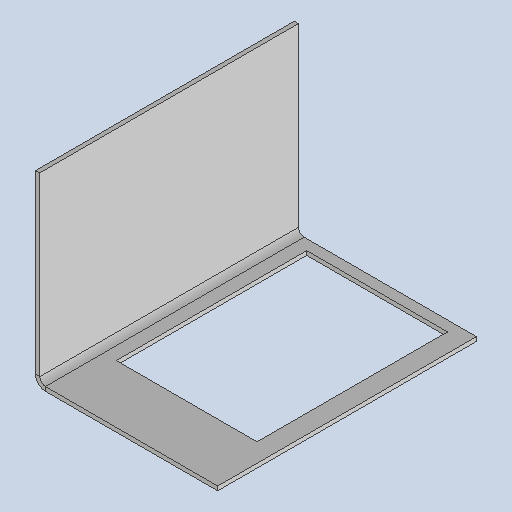
# Autodesk Inventor part: KND-1652 DrSysB Central tube wall 01
Saved by Autodesk Inventor 2026.2 (Build 302298000, 298)
## iProperties
Created: 2025-06-24
Part Number: KND-1652 DrSysB Central tube wall 01
Material: Stainless Steel
Document SubType Name: Sheet Metal
Designer: admin
Mass: 193.508 g
Surface Area: 260.557 cm^2
Volume: 24.1885 cm^3
Density: 8 g/cm^3
Flat Pattern Width: 17.4202 cm
Flat Pattern Length: 12.5 cm
Flat Pattern Area: 217.752 cm^2
Sheet Metal Rule: AISI304 2mm Die16
Sheet Metal Width: 174,202 mm
Sheet Metal Length: 125,000 mm
Sheet Metal Area: 21775,249 mm^2
Appearance: Default
Author: user
Autodesk Inventor part; units mm, degrees
ref_plane "YZ Plane" through (0, 0, 0) normal (1, 0, 0) x (0, 1, 0)
ref_plane "XZ Plane" through (0, 0, 0) normal (0, 1, 0) x (-1, 0, 0)
ref_plane "XY Plane" through (0, 0, 0) normal (0, 0, 1) x (1, 0, 0)
sketch "Sketch1" plane through (0, 0, 0) normal (0, 0, 1) x (1, 0, 0)
  line L0 (-44, -62.5) -> (44, -62.5)
  line L1 (44, -62.5) -> (44, 62.5)
  line L2 (44, 62.5) -> (-44, 62.5)
  line L3 (-44, 62.5) -> (-44, -62.5)
  line L4 (-44, -62.5) -> (44, 62.5) construction
  line L5 (44, -62.5) -> (-44, 62.5) construction
  line L6 (35, 57.5) -> (-33, 57.5)
  line L7 (-33, 57.5) -> (-33, -34.5)
  line L8 (-33, -34.5) -> (35, -34.5)
  line L9 (35, -34.5) -> (35, 57.5)
  point P0 (0, 0)
  dimension "d154" = 88
  dimension "d155" = 125
  dimension "d185" = 68
  dimension "d186" = 92
  dimension "d187" = 11
  dimension "d188" = 9
  dimension "d190" = 5
  measures "d154" distance of L1.end L2.end
  measures "d155" distance of L0.end L1.end
  measures "d185" distance of L8.end L7.end
  measures "d186" distance of L7.end L6.end
  measures "d187" distance between parallel lines of L7 L3
  measures "d188" distance between parallel lines of L1 L9
  measures "d190" distance between parallel lines of L6 L2
extrude "Plate5" add sketch "Sketch1" along normal blind 2
sketch "Sketch7" plane through (-42, -62.5, 0) normal (-1, 0, 0) x (0, -1, 0)
  line L0 (-125, 0) -> (0, 0)
  line L1 (0, 0) -> (0, 90)
  line L2 (0, 90) -> (-125, 90)
  line L3 (-125, 90) -> (-125, 0)
  constraints: 6 end point, 1 horizontal, 1 perpendicular, 1 vertical
edge flange "Flange3" height 90 angle 90 thickness 2 bend radius 2.75 thickness toward (-1, 0, 0) relief round relief width 2 relief depth 1 edges at (-44, 0, 2) wall of the first edge with corners at (-42, 62.5, 0) (-42, -62.5, 0) (-42, -62.5, 90) (-42, 62.5, 90)
bend "Bend3"
corner "Corner3"
sketch "Sketch9" plane through (-44, -62.5, 90) normal (-1, 0, 0) x (0, 0, 1)
  line L0 (-27.375, 69.75) -> (-57.875, 69.75)
  line L1 (-57.875, 69.75) -> (-57.875, 100.25)
  line L2 (-57.875, 100.25) -> (-27.375, 100.25)
  line L3 (-27.375, 100.25) -> (-27.375, 69.75)
  line L4 (-27.375, 69.75) -> (-57.875, 100.25) construction
  line L5 (-57.875, 69.75) -> (-27.375, 100.25) construction
  circle A0 centre (-19.625, 62) radius 2.5
  circle A1 centre (-65.625, 62) radius 2.5
  circle A2 centre (-65.625, 108) radius 2.5
  circle A3 centre (-19.625, 108) radius 2.5
  circle A4 centre (-42.625, 85) radius 32.5269 construction
  line L6 (-57.875, 69.75) -> (-65.625, 62) construction
  line L7 (-17.125, 59.5) -> (-68.125, 59.5) construction
  line L8 (-68.125, 59.5) -> (-68.125, 110.5) construction
  line L9 (-68.125, 110.5) -> (-17.125, 110.5) construction
  line L10 (-17.125, 110.5) -> (-17.125, 59.5) construction
  line L11 (-17.125, 59.5) -> (-68.125, 110.5) construction
  line L12 (-68.125, 59.5) -> (-17.125, 110.5) construction
  line L13 (-85.25, 125) -> (0, 125) projected
  line L14 (-42.625, 125) -> (-42.625, 85) construction
  circle A5 centre (-65.625, 108) radius 10.9602 construction
  line L15 (-19.625, 62) -> (-65.625, 62) construction
  line L16 (-65.625, 62) -> (-65.625, 108) construction
  line L17 (-65.625, 108) -> (-19.625, 108) construction
  line L18 (-19.625, 108) -> (-19.625, 62) construction
  line L19 (-19.625, 62) -> (-65.625, 108) construction
  line L20 (-65.625, 62) -> (-19.625, 108) construction
  point P0 (-90, 62.5)
  point P1 (-104.8197, 150.8767)
  point P2 (-104.8197, 150.8767)
  dimension "d181" = 21.9203
  dimension "d174" = 30.5
  dimension "d175" = 30.5
  dimension "d176" = 5
  dimension "d179" = 40
  dimension "d180" = 51
  dimension "d184" = 46
  constraints: 40 end point, 7 midpoint, 6 parallel, 5 centre point, 5 point on line, 4 point on circle, 3 equal radius, 3 horizontal, 3 perpendicular, 2 coincident, 1 tangent, 1 vertical, 3 other
  measures "d174" distance of L3.end L1.start
  measures "d175" distance of L1.start L1.end
  measures "d176" diameter of A0
  measures "d179" distance from line of L14.end L13
  measures "d180" distance of L7.end L8.end
  measures "d184" distance of L17.end L15.start
cut "Cut2" [suppressed]
body "Solid3"
